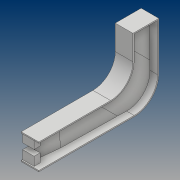
# Autodesk Inventor part: 軌道
Saved by Autodesk Inventor 2018 (Build 220112000, 112)
## iProperties
Created: 2020-11-30
Part Number: 軌道
Material: 一般
Document SubType Name: Modeling
Designer: 88697
Density: 1 g/cm^3
Appearance: 預設
Mass: 155.793 g
Surface Area: 478.827 cm^2
Volume: 155.793 cm^3
Author: 88697
Autodesk Inventor part; units mm, degrees
sketch "草圖2" plane through (0, 0, 0) normal (1, 0, 0) x (0, 1, 0)
  line L0 (0, 0) -> (150, 0)
  line L1 (150, 0) -> (150, -40)
  line L2 (150, -40) -> (0, -40)
  line L3 (0, -40) -> (0, 0)
  line L4 (150, -40) -> (110, -40)
  line L5 (110, -40) -> (110, 80)
  line L6 (110, 80) -> (150, 80)
  line L7 (150, 80) -> (150, -40)
  dimension "d2" = 40
  dimension "d3" = 150
  dimension "d4" = 40
  dimension "d5" = 120
  constraints: 16 end point, 4 parallel, 2 horizontal, 2 perpendicular
  measures "d2" distance of L2.end L0.start
  measures "d3" distance of L1.end L2.end
  measures "d4" distance of L5.end L6.end
  measures "d5" distance of L4.end L5.end
extrude "擠出1" add sketch "草圖2" along normal blind 10
fillet "圓角1" radius 40 2 edges at (5, 150, -40) (5, 110, 0)
sketch "草圖3" plane through (10, 0, 0) normal (1, 0, 0) x (0, 0, -1)
  arc A0 (0, 70) -> (-40, 110) centre (-40, 70) ccw projected
  arc A1 (40, 110) -> (0, 150) centre (0, 110) ccw projected
  line L0 (-40, 70) -> (0, 110) construction
  point P0 (0, 0)
  constraints: 2 coincident, 2 end point
sketch "草圖4" plane through (0, 0, 0) normal (-1, 0, 0) x (0, 0, 1)
  arc A0 (40, 110) -> (0, 70) centre (40, 70) ccw projected
  point P0 (0, 0)
  constraints: 1 coincident
ref_plane "工作平面1" through (10, 70, 40) normal (0, -0.7071068, -0.7071068) x (-1, 0, 0)
sketch "草圖5" plane through (10, 70, 40) normal (0, -0.7071068, -0.7071068) x (-1, 0, 0)
  line L0 (0, 40) -> (0, 28.2843) projected
  line L1 (0, 84.8528) -> (0, 96.5685) projected
  line L2 (0, 40) -> (0, 96.5685)
  line L3 (0, 96.5685) -> (-5.9456, 96.5685)
  line L4 (-5.9456, 96.5685) -> (0, 40)
  point P0 (10, -21.2132)
  dimension "d9" = 6
  constraints: 6 end point, 1 perpendicular, 1 vertical
  measures "d9" angle of L2 L4
ref_plane "工作平面2" through (10, 98.2843, 11.7157) normal (-0.9911739, 0.0156914, -0.1316365) x (0.1045285, 0.7032332, -0.7032332)
sketch "草圖7" plane through (10, 0, 0) normal (1, 0, 0) x (0, 0, -1)
  arc A0 (40, 110) -> (0, 150) centre (0, 110) ccw projected
  line L0 (40, 110) -> (40, 0) projected
  line L1 (40, 0) -> (0, 0) projected
  line L2 (0, 0) -> (0, 70) projected
  arc A1 (0, 70) -> (-40, 110) centre (-40, 70) ccw projected
  line L3 (-40, 110) -> (-80, 110) projected
  line L4 (-80, 110) -> (-80, 150) projected
  line L5 (-80, 150) -> (0, 150) projected
  arc A2 (0, 70) -> (-40, 110) centre (-40, 70) ccw projected
  line L6 (-11.7157, 98.2843) -> (28.2843, 138.2843)
  arc A3 (40, 110) -> (0, 150) centre (0, 110) ccw projected
  constraints: 4 point on circle, 2 end point
extrude "擠出4" add sketch "草圖7" against normal up to surface contours L0 L1 L2 A1 L6 A0 surface through (10, 98.2843, 11.7157) normal (-0.9911739, 0.0156914, -0.1316365)
ref_plane "工作平面6" through (15.9456, 138.2843, -28.2843) normal (-0.9918164, 0.1258338, -0.0215897) x (-0.1045285, -0.7032332, 0.7032332)
extrude "擠出5" add sketch "草圖7" against normal up to surface contours L6 A1 L3 L4 L5 A0 surface through (15.9456, 138.2843, -28.2843) normal (-0.9918164, 0.1258338, -0.0215897)
ref_plane "工作平面8" through (0, -50, -40) normal (0, -1, 0) x (1, 0, 0)
sketch "草圖9" plane through (0, -50, -40) normal (0, -1, 0) x (1, 0, 0)
  line L0 (0, 40) -> (10, 40)
  line L1 (10, 40) -> (10, 0)
  line L2 (10, 0) -> (0, 0)
  line L3 (0, 0) -> (0, 40)
  dimension "d53" = 10
  dimension "d54" = 40
  constraints: 8 end point, 2 parallel, 1 horizontal, 1 perpendicular
  measures "d53" distance of L1.end L2.end
  measures "d54" distance of L2.end L0.start
loft "斷面混成5" add profiles "草圖9" section 2 edges at (0, 0, -20) (7.6562, 0, -40) (12.6562, 0, -20) (5, 0, 0)
sketch "草圖10" plane through (0, 0, 0) normal (-1, 0, 0) x (0, 0, 1)
  arc A0 (0, 150) -> (-40, 110) centre (0, 110) ccw projected
  line L0 (0, 150) -> (80, 150) projected
  line L1 (80, 150) -> (80, 110) projected
  line L2 (80, 110) -> (40, 110) projected
  arc A1 (40, 110) -> (0, 70) centre (40, 70) ccw projected
  line L3 (0, 70) -> (0, -50) projected
  line L4 (0, -50) -> (-40, -50) projected
  line L5 (-40, -50) -> (-40, 110) projected
  arc A2 (0, 152) -> (-42, 110) centre (0, 110) ccw
  line L6 (0, 152) -> (82, 152)
  line L7 (82, 152) -> (82, 108)
  line L8 (82, 108) -> (40, 108)
  arc A3 (40, 108) -> (2, 70) centre (40, 70) ccw
  line L9 (2, 70) -> (2, -52)
  line L10 (2, -52) -> (-42, -52)
  line L11 (-42, -52) -> (-42, 110)
  point P0 (0, 0)
  dimension "d60" = 2
  constraints: 12 end point, 4 point on circle, 2 centre point, 7 other
  measures "d60" distance between parallel lines of L5 L11
extrude "擠出6" add sketch "草圖10" against normal blind 30
sketch "草圖11" plane through (30, 0, 0) normal (1, 0, 0) x (0, 0, -1)
  line L0 (0, -50) -> (0, 70) projected
  line L1 (-2, -52) -> (42, -52) projected
  line L2 (0, -50) -> (40, -50)
  line L3 (40, -50) -> (40, -52)
  line L4 (40, -52) -> (0, -52)
  line L5 (0, -52) -> (0, -50)
  line L6 (40, 110) -> (40, -50) projected
  point P0 (0, 0)
  constraints: 8 end point, 2 parallel, 1 collinear, 1 horizontal, 1 perpendicular, 1 point on line
extrude "擠出7" cut sketch "草圖11" against normal blind 30
sketch "草圖13" plane through (0, -50, 0) normal (0, -1, 0) x (1, 0, 0)
  line L0 (11.1082, 0) -> (10, 0) projected
  line L1 (10, 0) -> (20, 0)
  line L2 (20, 0) -> (20, -15)
  line L3 (20, -15) -> (10, -15)
  line L4 (10, -15) -> (10, 0)
  line L5 (10, 0) -> (10, -40) projected
  line L6 (10, -40) -> (20, -40)
  line L7 (20, -40) -> (20, -25)
  line L8 (20, -25) -> (10, -25)
  line L9 (10, -25) -> (10, -40)
  point P0 (0, 0)
  point P1 (10.4322, 0)
  dimension "d65" = 10
  dimension "d66" = 15
  dimension "d67" = 10
  dimension "d68" = 10
  constraints: 16 end point, 4 parallel, 2 horizontal, 2 perpendicular
  measures "d65" distance between parallel lines of L3 L8
  measures "d66" distance between parallel lines of L6 L8
  measures "d67" distance between parallel lines of L4 L2
  measures "d68" distance between parallel lines of L5 L7
extrude "擠出8" add sketch "草圖13" against normal blind 10
sketch "草圖14" plane through (30, 0, 0) normal (1, 0, 0) x (0, 0, -1)
  line L0 (-80, 110) -> (-80, 150) projected
  line L1 (-40, 110) -> (-80, 110) projected
  line L2 (-80, 150) -> (-65, 150)
  line L3 (-65, 150) -> (-65, 110)
  line L4 (-65, 110) -> (-80, 110)
  line L5 (-80, 110) -> (-80, 150)
  point P0 (0, 0)
  dimension "d71" = 15
  constraints: 8 end point, 2 parallel, 1 horizontal, 1 perpendicular, 1 point on line
  measures "d71" distance between parallel lines of L0 L3
extrude "擠出9" cut sketch "草圖14" against normal through all
ref_plane "工作平面9" through (10, -50, -20) normal (0, 0, 1) x (1, 0, 0)
sketch "草圖16" plane through (20, -50, 0) normal (1, 0, 0) x (0, 0, -1)
  line L0 (25, 10) -> (40, 10) projected
  line L1 (15, 0) -> (25, 0) projected
  line L2 (25, 10) -> (15, 10)
  line L3 (15, 10) -> (15, 0)
  line L4 (15, 0) -> (25, 0)
  line L5 (25, 0) -> (25, 10)
  point P0 (0, 50)
  constraints: 8 end point, 2 parallel, 1 horizontal, 1 perpendicular
extrude "擠出11" cut sketch "草圖16" against normal up to surface (20 mm away)
chamfer "倒角2" distance 0.5 angle 45 2 edges at (0, -45, -15) (0, -45, -25)
fillet "圓角4" radius 500 1 edges at (12.9728, 118.2843, -8.2843)
